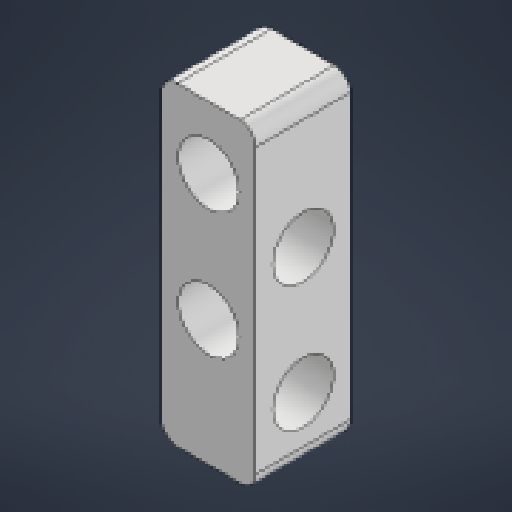
# Autodesk Inventor part: 3DPRINT,NUT-BLOCK
Saved by Autodesk Inventor 2026.1 (Build 301233020, 233B)
## iProperties
Created: 2026-04-01
Part Number: 3DPRINT,NUT-BLOCK
Material: Nylon 6/6
Document SubType Name: Modeling
Designer: Owen L
Mass: 4.08022 g
Surface Area: 26.3593 cm^2
Volume: 3.61082 cm^3
Density: 1.13 g/cm^3
Appearance: Smooth - Black
Author: Owen L
Autodesk Inventor part; units mm, degrees
ref_plane "YZ Plane" through (0, 0, 0) normal (1, 0, 0) x (0, 1, 0)
ref_plane "XZ Plane" through (0, 0, 0) normal (0, 1, 0) x (-1, 0, 0)
ref_plane "XY Plane" through (0, 0, 0) normal (0, 0, 1) x (1, 0, 0)
sketch "Sketch1" plane through (0, 0, 0) normal (1, 0, 0) x (0, 1, 0)
  line L0 (15.875, 6.35) -> (-15.875, 6.35)
  line L1 (-15.875, 6.35) -> (-15.875, -6.35)
  line L2 (-15.875, -6.35) -> (15.875, -6.35)
  line L3 (15.875, -6.35) -> (15.875, 6.35)
  line L4 (15.875, 6.35) -> (-15.875, -6.35) construction
  line L5 (-15.875, 6.35) -> (15.875, -6.35) construction
  point P0 (0, 0)
  dimension "d0" = 31.75
  dimension "d1" = 12.7
  constraints: 12 end point, 2 midpoint, 2 parallel, 1 horizontal, 1 perpendicular
  measures "d0" distance of L2.end L1.end
  measures "d1" distance of L1.end L0.end
extrude "Extrusion1" add sketch "Sketch1" along normal blind 12.7
sketch "Sketch2" plane through (12.7, 0, 0) normal (1, 0, 0) x (0, 0, -1)
  line L0 (6.35, 15.875) -> (-6.35, 15.875) projected
  point P0 (0, 0)
  point P1 (0, -9.525)
  point P2 (0, 3.175)
  dimension "d4" = 12.7
  dimension "d5" = 12.7
  constraints: 2 vertical alignment
  measures "d4" distance of point (0, -9.525) point (0, 3.175)
  measures "d5" distance from line of L0 point (0, 3.175)
hole "Hole1" at (12.7, -9.525, 0) at (12.7, 3.175, 0) direction (-1, 0, 0) diameter 6.096 depth 25.4 tip angle 118
sketch "Sketch3" plane through (0, -15.875, 6.35) normal (0, 0, 1) x (1, 0, 0)
  line L0 (0, 31.75) -> (12.7, 31.75) projected
  point P0 (0, 15.875)
  point P1 (6.35, 25.4)
  point P2 (6.35, 12.7)
  point P3 (6.35, 31.75)
  dimension "d13" = 12.7
  dimension "d14" = 6.35
  constraints: 2 vertical alignment, 1 midpoint
  measures "d13" distance of point (6.35, 25.4) point (6.35, 12.7)
  measures "d14" distance from line of L0 point (6.35, 25.4)
hole "Hole2" at (6.35, 9.525, 6.35) at (6.35, -3.175, 6.35) direction (0, 0, -1) diameter 6.096 depth 25.4 tip angle 118
fillet "Fillet1" radius 1.5875 4 edges at (12.7, -15.875, 0) (0, -15.875, 0) (12.7, 15.875, 0) (0, 15.875, 0)
body "Solid1"
